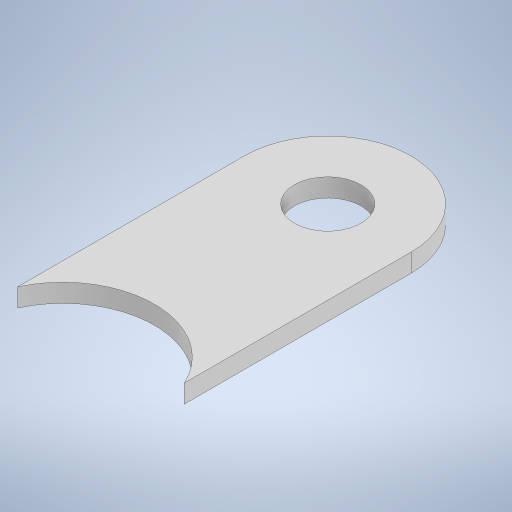
# Autodesk Inventor part: ギアプレートupper_upper
Saved by Autodesk Inventor 2024.1 (Build 281209000, 209)
## iProperties
Created: 2024-04-01
Part Number: ギアプレートupper_upper
Material: 一般
Document SubType Name: Modeling
Designer: hibik
Density: 1 g/cm^3
Appearance: 既定
Author: hibik
Autodesk Inventor part; units mm, degrees
ref_plane "YZ Plane" through (0, 0, 0) normal (1, 0, 0) x (0, 1, 0)
ref_plane "XZ Plane" through (0, 0, 0) normal (0, 1, 0) x (-1, 0, 0)
ref_plane "XY Plane" through (0, 0, 0) normal (0, 0, 1) x (1, 0, 0)
sketch "スケッチ1" plane through (0, 0, 0) normal (0, 1, 0) x (-1, 0, 0)
  line L0 (25, 0) -> (-25, 0)
  line L1 (-25, 0) -> (-25, -159)
  line L2 (-25, -159) -> (25, -159)
  line L3 (25, -159) -> (25, 0)
  circle A0 centre (0, 0) radius 25
  circle A1 centre (0, 0) radius 57 construction
  circle A2 centre (0, -79.5) radius 22.5 construction
  circle A3 centre (0, 0) radius 75 construction
  circle A4 centre (0, -79.5) radius 10
  circle A5 centre (0, 0) radius 10
  circle A6 centre (0, -159) radius 10
  circle A7 centre (0, -159) radius 57 construction
  circle A8 centre (0, -159) radius 25
  circle A9 centre (0, -79.5) radius 27.5
  point P0 (25, -90.9564)
  point P1 (-25, -90.9564)
  dimension "d0" = 114
  dimension "d1" = 45
  dimension "d2" = 150
  dimension "d3" = 20
  dimension "d4" = 20
  dimension "d5" = 50
  dimension "d8" = 20
  dimension "d13" = 55
  constraints: 9 centre point, 9 coincident, 8 end point, 3 tangent, 2 midpoint, 2 parallel, 2 vertical alignment, 1 equal radius, 1 horizontal, 1 perpendicular, 3 other
  measures "d0" diameter of A1
  measures "d1" diameter of A2
  measures "d2" diameter of A3
  measures "d3" diameter of A4
  measures "d4" diameter of A5
  measures "d5" distance of L1.end L2.end
  measures "d8" diameter of A6
  measures "d13" diameter of A9
extrude "押し出し1" add sketch "スケッチ1" along normal blind 5.5 contours L3 A8 L1 A9 | A8 L2 A6 | L2 A6 A8
